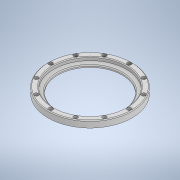
# Autodesk Inventor part: KF160_adaptor
Saved by Autodesk Inventor 2021 (Build 250183000, 183)
## iProperties
Created: 2024-01-23
Part Number: KF160_adaptor
Material: Generic
Document SubType Name: Modeling
Designer: Sebastián
Density: 1 g/cm^3
Appearance: Default
Author: Sebastián
Autodesk Inventor part; units mm, degrees
ref_plane "YZ Plane" through (0, 0, 0) normal (1, 0, 0) x (0, 1, 0)
ref_plane "XZ Plane" through (0, 0, 0) normal (0, 1, 0) x (-1, 0, 0)
ref_plane "XY Plane" through (0, 0, 0) normal (0, 0, 1) x (1, 0, 0)
sketch "Sketch1" plane through (0, 0, 0) normal (1, 0, 0) x (0, 1, 0)
  line L0 (0, 84.5) -> (5, 84.5)
  line L1 (5, 84.5) -> (7.8671, 95.2)
  line L2 (7.8671, 95.2) -> (17, 95.2)
  line L3 (5, 84.5) -> (5, 129.2846) construction
  line L4 (0, 84.5) -> (0, 110.2)
  line L5 (0, 110.2) -> (17, 110.2)
  line L6 (17, 110.2) -> (17, 95.2)
  line L7 (-3.4, 0) -> (20.4, 0) projected
  point P0 (0, 0)
  dimension "d0" = 15
  dimension "d1" = 95.2
  dimension "d3" = 84.5
  dimension "d4" = 5
  dimension "d5" = 12
  dimension "d7" = 15
  constraints: 14 end point, 3 parallel, 2 perpendicular, 1 vertical
  measures "d0" angle of L3 L1
  measures "d1" vertical distance of point (0, 0) L2.end
  measures "d3" vertical distance of point (0, 0) L0.end
  measures "d4" distance of L0.end L0.start
  measures "d5" horizontal distance of L2.end L0.end
  measures "d7" distance of L5.end L2.end
revolve "Revolution1" add sketch "Sketch1" angle 360 about axis through (0, -10, 0) along (0, 1, 0)
sketch "Sketch2" plane through (0, 0, 0) normal (0, -1, 0) x (1, 0, 0)
  circle A0 centre (0, 0) radius 95.2 construction
  circle A1 centre (0, 0) radius 110.2 construction
  circle A2 centre (0, -103) radius 5.25
  dimension "d9" = 10.5
  dimension "d10" = 103
  constraints: 1 centre point
  measures "d9" diameter of A2
  measures "d10" distance of point (0, 0) A2.centre
extrude "Extrusion1" cut sketch "Sketch2" against normal through all
pattern_circular "Circular Pattern1" count 12 over 360 about axis through (0, -10, 0) along (0, 1, 0) of "Extrusion1"
chamfer "Chamfer1" distance 2 angle 45 3 edges at (0, 5, -84.5) (0, 17, -95.2) (0, 17, -110.2)
body "Solid1"
